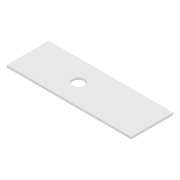
# Autodesk Inventor part: 00_Microscopeslide
Saved by Autodesk Inventor 2019.4 (Build 234330000, 330)
## iProperties
Created: 2020-07-07
Part Number: 00_Microscopeslide
Material: Generic
Document SubType Name: Modeling
Designer: diederichbenedict
Density: 1 g/cm^3
Appearance: Polycarbonate - Clear
Author: diederichbenedict
Autodesk Inventor part; units mm, degrees
ref_plane "YZ Plane" through (0, 0, 0) normal (1, 0, 0) x (0, 1, 0)
ref_plane "XZ Plane" through (0, 0, 0) normal (0, 1, 0) x (-1, 0, 0)
ref_plane "XY Plane" through (0, 0, 0) normal (0, 0, 1) x (1, 0, 0)
sketch "Sketch1" plane through (0, 0, 0) normal (0, 1, 0) x (-1, 0, 0)
  line L0 (0, 0) -> (-75.4, 0)
  line L1 (-75.4, 0) -> (-75.4, 25.5)
  line L2 (-75.4, 25.5) -> (0, 25.5)
  line L3 (0, 25.5) -> (0, 0)
  dimension "d0" = 75.4
  dimension "d1" = 25.5
  constraints: 8 end point, 2 parallel, 1 horizontal, 1 perpendicular
  measures "d0" distance of L1.end L2.end
  measures "d1" distance of L0.end L1.end
extrude "Extrusion1" add sketch "Sketch1" along normal blind 1.3
sketch "Sketch6" plane through (0, 1.3, 0) normal (0, 1, 0) x (1, 0, 0)
  line L0 (75.4, 0) -> (0, 0) projected
  line L1 (0, 0) -> (0, -25.5) projected
  line L2 (0, -25.5) -> (75.4, -25.5) projected
  line L3 (75.4, -25.5) -> (75.4, 0) projected
  circle A0 centre (30.7, -12.75) radius 3.5
  dimension "d20" = 7
  dimension "d24" = 30.7
  constraints: 1 centre point
  measures "d20" diameter of A0
  measures "d24" distance from line of A0.centre L1
extrude "Extrusion6" cut sketch "Sketch6" against normal blind 10 contours A0
body "Solid1"
